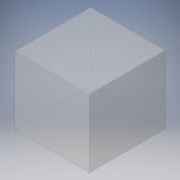
# Autodesk Inventor part: maxAllowedVolumeForDriving
Saved by Autodesk Inventor 2016 SP1 (Build 200210100, 210)
## iProperties
Created: 2016-01-26
Part Number: maxAllowedVolumeForDriving
Material: Polycarbonate, Clear
Document SubType Name: Modeling
Designer: steele
Density: 1.2 g/cm^3
Appearance: Polycarbonate - Clear
Author: steele
Autodesk Inventor part; units mm, degrees
ref_plane "YZ Plane" through (0, 0, 0) normal (1, 0, 0) x (0, 1, 0)
ref_plane "XZ Plane" through (0, 0, 0) normal (0, 1, 0) x (-1, 0, 0)
ref_plane "XY Plane" through (0, 0, 0) normal (0, 0, 1) x (1, 0, 0)
sketch "Sketch1" plane through (0, 0, 0) normal (0, 1, 0) x (-1, 0, 0)
  line L0 (755.65, 768.35) -> (-755.65, 768.35)
  line L1 (-755.65, 768.35) -> (-755.65, -768.35)
  line L2 (-755.65, -768.35) -> (755.65, -768.35)
  line L3 (755.65, -768.35) -> (755.65, 768.35)
  line L4 (755.65, 768.35) -> (-755.65, -768.35) construction
  line L5 (-755.65, 768.35) -> (755.65, -768.35) construction
  point P0 (0, 0)
  dimension "d0" = 1536.7
  dimension "d1" = 1511.3
  constraints: 12 end point, 2 midpoint, 2 parallel, 1 horizontal, 1 perpendicular
  measures "d0" distance of L2.end L0.start
  measures "d1" distance of L0.start L0.end
extrude "Extrusion1" add sketch "Sketch1" along normal blind 1371.6
equation "\"d0\" = maxVolumeLength"
equation "\"d1\" = maxVolumeWidth"
equation "\"d2\" = maxVolumeHeight"
equation "\"robotWidth\" = -robotLength + 0.5 * perimeter"
equation "\"robotLength\" = 774.7"
equation "\"maxVolumeHeight\" = 1371.6"
equation "\"perimeter\" = 3048"
equation "\"maxVolumeLength\" = 1536.7"
equation "\"maxVolumeWidth\" = 1511.3"
body "Solid1"
